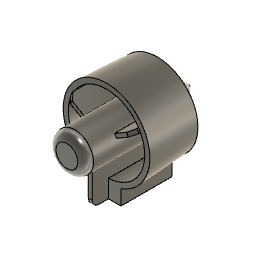
Water jet adapter (Autodesk Fusion 360 archive; units mm, degrees)
design "2216 Thruster EK"
Autodesk Fusion 360 part; units mm, degrees
sketch "Sketch1" plane through (0, 0, 0) normal (0, 1, 0) x (1, 0, 0) in component "thruster"
  circle A0 centre (0, 0) radius 15.65
  circle A1 centre (0, 0) radius 31.665
  circle A2 centre (0, 0) radius 35.935
  line L0 (-12.025, 37.3633) -> (12.025, 37.3633)
  line L1 (12.025, 37.3633) -> (12.025, 46.3633)
  line L2 (12.025, 46.3633) -> (-12.025, 46.3633)
  line L3 (-12.025, 46.3633) -> (-12.025, 37.3633)
  line L4 (0, 37.3633) -> (0, 46.3633) construction
  line L5 (0, 0) -> (0, 35.935) construction
  line L6 (-12.025, 33.8633) -> (-12.025, 37.3633)
  line L7 (-12.025, 37.3633) -> (12.025, 37.3633)
  line L8 (0, 37.3633) -> (0, 35.935) construction
  line L9 (12.025, 37.3633) -> (12.025, 33.8633)
  line L10 (-1.6, 12.65) -> (1.6, 12.65)
  line L11 (1.6, 12.65) -> (1.6, 34.665)
  line L12 (1.6, 34.665) -> (-1.6, 34.665)
  line L13 (-1.6, 34.665) -> (-1.6, 12.65)
  line L14 (0, 34.665) -> (0, 12.65) construction
  line L15 (0, 15.65) -> (6.1673, 15.65) construction
  line L16 (0, 31.665) -> (7.6621, 31.665) construction
  line L17 (-29.2208, -18.7181) -> (-10.1552, -7.7106)
  line L18 (-10.1552, -7.7106) -> (-11.7552, -4.9394)
  line L19 (-11.7552, -4.9394) -> (-30.8208, -15.9469)
  line L20 (-30.8208, -15.9469) -> (-29.2208, -18.7181)
  line L21 (30.8208, -15.9469) -> (11.7552, -4.9394)
  line L22 (11.7552, -4.9394) -> (10.1552, -7.7106)
  line L23 (10.1552, -7.7106) -> (29.2208, -18.7181)
  line L24 (29.2208, -18.7181) -> (30.8208, -15.9469)
  line L25 (-1.6, 34.665) -> (1.6, 34.665)
  line L26 (1.6, 34.665) -> (1.6, 46.3633)
  line L27 (1.6, 46.3633) -> (-1.6, 46.3633)
  line L28 (-1.6, 46.3633) -> (-1.6, 34.665)
  dimension "d1" = 31.3
  dimension "d2" = 4.27
  dimension "d3" = 71.87
  dimension "d4" = 24.05
  dimension "d5" = 9
  dimension "d6" = 3.5
  dimension "d7" = 24.05
  dimension "d10" = 3.2
  dimension "d11" = 3
  dimension "d12" = 3
  dimension "d14" = 360
  constraint coincident A0.centre A1.centre
  constraint concentric A0 A2
  constraint horizontal L0
  constraint vertical L1
  constraint horizontal L2
  constraint vertical L3
  constraint midpoint L0 L4.start
  constraint midpoint L2 L4.end
  constraint coincident A2 L5.end
  constraint parallel L4 L5
  constraint coincident A2 L6.start
  constraint vertical L6
  constraint perpendicular L6 L7
  constraint midpoint L7 L4.start
  constraint perpendicular L7 L8
  constraint collinear L5 L8
  constraint coincident A2 L9.end
  constraint perpendicular L7 L9
  constraint coincident L0 L3.end
  constraint coincident L0.start L3.end
  constraint horizontal L10
  constraint vertical L11
  constraint horizontal L12
  constraint vertical L13
  constraint midpoint L12 L14.start
  constraint midpoint L10 L14.end
  constraint collinear L5 L14
  constraint coincident A0 L15.start
  constraint coincident L5 L15.start
  constraint tangent A0 L15
  constraint coincident L14 L16.start
  constraint coincident A1 L16.start
  constraint tangent A1 L16
  constraint horizontal L25
  constraint vertical L26
  constraint horizontal L27
  constraint vertical L28
  constraint coincident L2 L26.end
  constraint coincident L11.end L26
  measures "d1" diameter of A0
  measures "d2" distance of A1 A2
  measures "d3" diameter of A2
  measures "d4" distance of L1.end L2.end
  measures "d5" distance of L0.end L1.end
  measures "d6" distance of L6.start L0.start
  measures "d7" distance of L0.start L0.end
  measures "d10" distance of L11.end L12.end
  measures "d11" distance of L10 L15
  measures "d12" distance of L12 L16
extrude "Extrude1" add sketch "Sketch1" along normal blind 42.22 contours A0 L10 L11 L13 L17 L18 L19 L21 L22 L23 | A0 L10 L11 L13 | A0 A1 L11 L13 | A0 A1 L21 L23 | A0 L21 L22 L23 | A1 L11 L12 L13 L25 | A0 L17 L18 L19 | A0 A1 L17 L19 | A2 L12 L25 L26 L28 | A2 L0 L7 L9 L26 | A2 L0 L7 L26 L28 | A2 L0 L6 L7 L28 | L0 L1 L2 L7 L26 | L0 L2 L7 L26 L27 L28 | L0 L2 L3 L7 L28 makes body 1 in component "thruster"
extrude "Extrude2" add sketch "Sketch1" against normal blind 32.92 contours A0 L10 L11 L13 L17 L18 L19 L21 L22 L23 | A0 L10 L11 L13 | A0 L21 L22 L23 | A0 L17 L18 L19 bodies 1 in component "thruster"
extrude "Extrude3" add sketch "Sketch1" against normal blind 13.49 contours A0 A1 L11 L13 | A1 L11 L12 L13 L25 | A2 L12 L25 L26 L28 | A2 L0 L7 L26 L28 | L0 L2 L7 L26 L27 L28 bodies 1 in component "thruster"
extrude "Extrude4" add sketch "Sketch1" against normal blind 5.98 contours A0 A1 L21 L23 | A0 A1 L17 L19 bodies 1 in component "thruster"
chamfer "Chamfer1" distance 4.772 angle 45 2 edges at (27.4227, -5.98, 15.8325) (-27.4227, -5.98, 15.8325) on bodies 1 in component "thruster"
fillet "Fillet1" radius 5.637 1 edges at (0, -13.49, -46.3633) on bodies 1 in component "thruster"
fillet "Fillet2" radius 6.572 1 edges at (-14.5909, -32.92, -5.6593) on bodies 1 in component "thruster"
ref_plane "WorkPlane1" through (0, 42.22, 0) normal (0, 1, 0) x (0, 0, 1) in component "thruster"
sketch "Sketch2" plane through (0, 42.22, 0) normal (0, 1, 0) x (1, 0, 0) in component "thruster"
  line L0 (12.025, 33.8633) -> (12.025, 46.3633)
  line L1 (12.025, 46.3633) -> (-12.025, 46.3633)
  line L2 (-12.025, 46.3633) -> (-12.025, 33.8633)
  arc A0 (-1.6, 35.8994) -> (-12.025, 33.8633) centre (0, 0) ccw
  line L3 (-1.6, 35.8994) -> (-1.6, 15.568)
  arc A1 (-1.6, 15.568) -> (-14.2823, -6.3984) centre (0, 0) ccw
  line L4 (-14.2823, -6.3984) -> (-28.1877, -14.4266)
  arc A2 (-28.1877, -14.4266) -> (-26.5877, -17.1979) centre (0, 0) ccw
  line L5 (-26.5877, -17.1979) -> (-12.6823, -9.1696)
  arc A3 (-12.6823, -9.1696) -> (12.6823, -9.1696) centre (0, 0) ccw
  line L6 (12.6823, -9.1696) -> (26.5877, -17.1979)
  arc A4 (26.5877, -17.1979) -> (28.1877, -14.4266) centre (0, 0) ccw
  line L7 (28.1877, -14.4266) -> (14.2823, -6.3984)
  arc A5 (14.2823, -6.3984) -> (1.6, 15.568) centre (0, 0) ccw
  line L8 (1.6, 15.568) -> (1.6, 35.8994)
  arc A6 (12.025, 33.8633) -> (1.6, 35.8994) centre (0, 0) ccw
  circle A7 centre (0, 0) radius 31.755
  circle A8 centre (0, 0) radius 33.575
  dimension "d27" = 1.82
  dimension "d28" = 67.15
  constraint concentric A0 A7
  constraint concentric A7 A8
  measures "d27" distance of A7 A8
  measures "d28" diameter of A8
loft "Loft1" add profiles "Sketch1", "Sketch2" section 1 contours A1 A2 L11 L13 L17 L19 L20 L21 L23 L24 L26 L28 | A1 L11 L12 L13 L25 | A1 L21 L23 L24 | A2 L12 L25 L26 L28 | A1 L17 L19 L20 section 2 contours L3 L8 A7 A8 | L3 L8 A7 A8 separate body makes body 2 in component "thruster"
sketch "Sketch3" plane through (0, 0, 0) normal (0, 1, 0) x (1, 0, 0) in component "thruster"
  circle A0 centre (0, 0) radius 35.935
  circle A1 centre (0, 0) radius 31.665
loft "Loft2" cut profiles "Sketch2", "Sketch3" section 1 contours L3 A1 L4 A2 L5 A3 L6 A4 L7 A5 L8 A7 | L3 A1 L4 A2 L5 A3 L6 A4 L7 A5 L8 A7 section 2 contours A1 bodies 2 in component "thruster"
sketch "Sketch4" plane through (0, 42.22, 0) normal (0, 1, 0) x (1, 0, 0) in component "thruster"
  line L0 (12.025, 33.8633) -> (12.025, 46.3633)
  line L1 (12.025, 46.3633) -> (-12.025, 46.3633)
  line L2 (-12.025, 46.3633) -> (-12.025, 33.8633)
  arc A0 (-1.6, 35.8994) -> (-12.025, 33.8633) centre (0, 0) ccw
  line L3 (-1.6, 35.8994) -> (-1.6, 15.568)
  arc A1 (-1.6, 15.568) -> (-14.2823, -6.3984) centre (0, 0) ccw
  line L4 (-14.2823, -6.3984) -> (-28.1877, -14.4266)
  arc A2 (-28.1877, -14.4266) -> (-26.5877, -17.1979) centre (0, 0) ccw
  line L5 (-26.5877, -17.1979) -> (-12.6823, -9.1696)
  arc A3 (-12.6823, -9.1696) -> (12.6823, -9.1696) centre (0, 0) ccw
  line L6 (12.6823, -9.1696) -> (26.5877, -17.1979)
  arc A4 (26.5877, -17.1979) -> (28.1877, -14.4266) centre (0, 0) ccw
  line L7 (28.1877, -14.4266) -> (14.2823, -6.3984)
  arc A5 (14.2823, -6.3984) -> (1.6, 15.568) centre (0, 0) ccw
  line L8 (1.6, 15.568) -> (1.6, 35.8994)
  arc A6 (12.025, 33.8633) -> (1.6, 35.8994) centre (0, 0) ccw
  circle A7 centre (0, 0) radius 31.755
  circle A8 centre (0, 0) radius 33.575
  line L9 (12.025, 33.8633) -> (12.025, 31.3477)
  line L10 (-12.025, 33.8633) -> (-12.025, 31.3477)
  constraint coincident L0.start A6.start
  constraint coincident A8 L9.end
  constraint parallel L0 L9
  constraint coincident L2.end A0.end
  constraint coincident A8 L10.end
  constraint parallel L2 L10
extrude "Extrude5" add sketch "Sketch4" against normal up to surface (42.22 mm away) contours L8 A6 A8 L9 | A0 L3 A8 L10 bodies 2 1 in component "thruster"
sketch "Sketch5" plane through (0, 42.22, 0) normal (0, 1, 0) x (1, 0, 0) in component "thruster"
  line L0 (12.025, 31.3477) -> (12.025, 46.3633)
  line L1 (12.025, 46.3633) -> (-12.025, 46.3633)
  line L2 (-12.025, 46.3633) -> (-12.025, 31.3477)
  arc A0 (-12.025, 31.3477) -> (12.025, 31.3477) centre (0, 0) ccw
  arc A1 (-1.6, 31.7147) -> (1.6, 31.7147) centre (0, 0) ccw
  line L3 (-1.6, 31.7147) -> (-1.6, 15.568)
  arc A2 (-1.6, 15.568) -> (-14.2823, -6.3984) centre (0, 0) ccw
  line L4 (-14.2823, -6.3984) -> (-28.1877, -14.4266)
  arc A3 (-28.1877, -14.4266) -> (-26.5877, -17.1979) centre (0, 0) ccw
  line L5 (-26.5877, -17.1979) -> (-12.6823, -9.1696)
  arc A4 (-12.6823, -9.1696) -> (12.6823, -9.1696) centre (0, 0) ccw
  line L6 (12.6823, -9.1696) -> (26.5877, -17.1979)
  arc A5 (26.5877, -17.1979) -> (28.1877, -14.4266) centre (0, 0) ccw
  line L7 (28.1877, -14.4266) -> (14.2823, -6.3984)
  arc A6 (14.2823, -6.3984) -> (1.6, 15.568) centre (0, 0) ccw
  line L8 (1.6, 15.568) -> (1.6, 31.7147)
  circle A7 centre (0, 0) radius 15.65
  circle A8 centre (0, 42.3633) radius 2.87
  line L9 (0, 46.3633) -> (0, 5.0666) construction
  dimension "d45" = 5.74
  dimension "d46" = 4
  constraint concentric A0 A7
  constraint coincident A4.end A7
  constraint midpoint L1 L9.start
  constraint perpendicular L1 L9
  constraint coincident A8.centre L9
  measures "d45" diameter of A8
  measures "d46" distance of L1 A8.centre
extrude "Extrude6" add sketch "Sketch5" along normal blind 26.29 separate body contours A2 A4 A6 A7 makes body 3 in component "thruster"
chamfer "Chamfer2" distance 15.004 angle 45 1 edges at (-14.5909, 68.51, 5.6593) on bodies 3 in component "thruster"
ref_plane "WorkPlane2" through (0, 17.1835, -46.3633) normal (0, 0, -1) x (-1, 0, 0) in component "thruster"
sketch "Sketch6" plane through (0, 17.1835, -46.3633) normal (0, 0, -1) x (1, 0, 0) in component "thruster"
  line L0 (1.6, 25.0365) -> (-1.6, 25.0365)
  line L1 (-1.6, 25.0365) -> (-1.6, 17.1835)
  line L2 (-1.6, 17.1835) -> (-12.025, 17.1835)
  line L3 (-12.025, 17.1835) -> (-12.025, -25.0365)
  line L4 (-12.025, -25.0365) -> (12.025, -25.0365)
  line L5 (12.025, -25.0365) -> (12.025, 17.1835)
  line L6 (12.025, 17.1835) -> (1.6, 17.1835)
  line L7 (1.6, 17.1835) -> (1.6, 25.0365)
  line L8 (-1.6, 17.1835) -> (1.6, 17.1835)
  line L9 (-10.025, -23.3865) -> (10.025, -23.3865) construction
  line L10 (10.025, -23.3865) -> (10.025, 15.5335) construction
  line L11 (10.025, 15.5335) -> (-10.025, 15.5335) construction
  line L12 (-10.025, 15.5335) -> (-10.025, -23.3865) construction
  circle A0 centre (-8.025, -21.3865) radius 2
  circle A1 centre (8.025, -21.3865) radius 2
  circle A2 centre (8.025, 13.5335) radius 2
  circle A3 centre (-8.025, 13.5335) radius 2
  dimension "d35" = 4
  dimension "d36" = 1.65
  dimension "d37" = 2
  dimension "d38" = 2
  dimension "d39" = 1.65
  dimension "d40" = 4
  dimension "d41" = 4
  dimension "d42" = 4
  constraint coincident L1.end L2.start
  constraint coincident L6.end L7.start
  constraint horizontal L9
  constraint vertical L10
  constraint horizontal L11
  constraint vertical L12
  constraint tangent L12 A0
  constraint tangent L9 A0
  constraint tangent L10 A1
  constraint tangent L9 A1
  constraint tangent L12 A3
  constraint tangent L11 A3
  constraint tangent L11 A2
  constraint tangent L10 A2
  measures "d35" diameter of A0
  measures "d36" distance of L4 L9
  measures "d37" distance of L3 L12
  measures "d38" distance of L5 L10
  measures "d39" distance of L2 L11
  measures "d40" diameter of A1
  measures "d41" diameter of A2
  measures "d42" diameter of A3
extrude "Extrude7" cut sketch "Sketch6" against normal blind 13.87 contours A0 | A1 | A2 | A3 bodies 2 in component "thruster"
extrude "Extrude8" add sketch "Sketch5" along normal blind 10 separate body contours A8 makes body 4 in component "thruster"
component "thruster" placed x (1, 0, 0) y (0, 1, 0) z (0, 0, 1) at (0, 0, 0)
